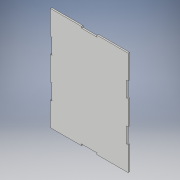
# Autodesk Inventor part: belakang
Saved by Autodesk Inventor 2017 (Build 210142000, 142)
## iProperties
Created: 2017-01-06
Part Number: belakang
Material: Generic
Document SubType Name: Modeling
Designer: Windows 8.1
Density: 1 g/cm^3
Appearance: Default
Author: Windows 8.1
Autodesk Inventor part; units mm, degrees
ref_plane "YZ Plane" through (0, 0, 0) normal (1, 0, 0) x (0, 1, 0)
ref_plane "XZ Plane" through (0, 0, 0) normal (0, 1, 0) x (-1, 0, 0)
ref_plane "XY Plane" through (0, 0, 0) normal (0, 0, 1) x (1, 0, 0)
sketch "Sketch1" plane through (0, 0, 0) normal (0, 0, 1) x (1, 0, 0)
  line L0 (60, 199.8) -> (60, 196.8)
  line L1 (60, 196.8) -> (90, 196.8)
  line L2 (90, 196.8) -> (90, 200)
  line L3 (90, 0) -> (90, 3)
  line L4 (90, 3) -> (60, 3)
  line L5 (60, 3) -> (60, 0)
  line L6 (149.9999, 200) -> (90, 200)
  line L7 (60, 199.8) -> (0, 199.8)
  line L8 (0, 0) -> (60, 0)
  line L9 (90, 0) -> (150, 0)
  line L10 (0, 153.2) -> (3, 153.2)
  line L11 (3, 153.2) -> (3, 123.2)
  line L12 (3, 123.2) -> (0, 123.2)
  line L13 (0, 76.6) -> (3, 76.6)
  line L14 (3, 76.6) -> (3, 46.6)
  line L15 (3, 46.6) -> (0, 46.6)
  line L16 (0, 199.8) -> (0, 153.2)
  line L17 (0, 123.2) -> (0, 76.6)
  line L18 (0, 46.6) -> (0, 0)
  line L19 (149.9999, 153.4) -> (146.9999, 153.4)
  line L20 (146.9999, 153.4) -> (146.9999, 123.4)
  line L21 (146.9999, 123.4) -> (149.9999, 123.4)
  line L22 (149.9999, 153.4) -> (149.9999, 200)
  line L23 (149.9999, 76.8) -> (147, 76.8)
  line L24 (147, 76.8) -> (147, 46.6)
  line L25 (147, 46.6) -> (150, 46.6)
  line L26 (150, 0) -> (150, 46.6)
  line L27 (149.9999, 76.8) -> (149.9999, 123.4)
  dimension "d1" = 200
  dimension "d2" = 150
  dimension "d4" = 30
  dimension "d6" = 3
  dimension "d26" = 30
  dimension "d27" = 60
  dimension "d28" = 60
  dimension "d29" = 30
  dimension "d30" = 30
  dimension "d31" = 3
  dimension "d32" = 3
  dimension "d34" = 3
  dimension "d35" = 3
  dimension "d36" = 46.6
  dimension "d37" = 46.6
  dimension "d38" = 46.6
  dimension "d39" = 46.6
  dimension "d40" = 46.6
  dimension "d41" = 46.6
  dimension "d44" = 3
  dimension "d45" = 3
  dimension "d46" = 3
  dimension "d47" = 3
  constraints: 56 end point, 30 perpendicular, 15 parallel, 3 horizontal, 2 point on line
  measures "d1" distance of L9.end L6.start
  measures "d2" distance of L6.start L7.end
  measures "d4" distance of L0.end L1.end
  measures "d6" distance of L0.start L0.end
  measures "d26" distance of L3.end L4.end
  measures "d27" distance of L8.start L5.end
  measures "d28" distance of L3.start L9.end
  measures "d29" distance of L10.end L11.end
  measures "d30" distance of L13.end L14.end
  measures "d31" distance of L11.end L12.end
  measures "d32" distance of L10.start L10.end
  measures "d34" distance of L14.end L15.end
  measures "d35" distance of L19.start L19.end
  measures "d36" distance of L7.end L10.start
  measures "d37" distance of L15.end L8.start
  measures "d38" distance of L12.end L13.start
  measures "d39" distance of L19.start L6.start
  measures "d40" distance of L23.start L21.end
  measures "d41" distance of L9.end L25.end
  measures "d44" distance of L24.end L25.end
  measures "d45" distance of L20.end L21.end
  measures "d46" distance of L4.end L5.end
  measures "d47" distance from line of L3.start L4
extrude "Extrusion1" add sketch "Sketch1" along normal blind 3
body "Solid1"
